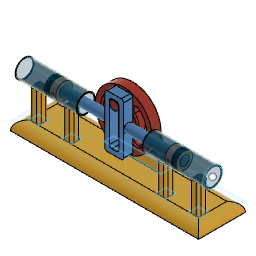
Scotch Yoke Mechanism (Autodesk Fusion 360 design; units mm, degrees)
Autodesk Fusion 360 part; units mm, degrees
sketch "base" plane through (0, 0, 0) normal (0, 0, 1) x (1, 0, 0) in component "Holder"
  line L0 (100, 0) -> (100, 25)
  line L1 (100, 0) -> (100, -25)
  line L2 (-100, 0) -> (-100, 25)
  line L3 (-100, 0) -> (-100, -25)
  line L4 (-100, 25) -> (100, 25)
  line L5 (-100, -25) -> (100, -25)
  dimension "d1" = 100
  dimension "d5" = 50
  constraint vertical L0
  constraint perpendicular L0 L4
  constraint perpendicular L1 L5
  measures "d1" distance of origin L0.start
  measures "d5" distance of L4 L5
extrude "Extrude1" add sketch "base" along normal blind 10 makes body 1 in component "Holder"
sketch "holders" plane through (0, 0, 10) normal (0, 0, 1) x (-1, 0, 0) in component "Holder"
  line L0 (100, -25) -> (100, 25)
  line L1 (100, 25) -> (-100, 25)
  line L2 (-100, 25) -> (-100, -25)
  line L3 (-100, -25) -> (100, -25)
  line L4 (30, -15) -> (-30, -15)
  line L5 (-30, -15) -> (-30, -5)
  line L6 (-30, -5) -> (30, -5)
  line L7 (30, -5) -> (30, -15)
  line L8 (90, 14.85) -> (80, 14.85)
  line L9 (80, 14.85) -> (80, 5)
  line L10 (80, 5) -> (90, 5)
  line L11 (55, 14.85) -> (45, 14.85)
  line L12 (45, 14.85) -> (45, 5)
  line L13 (45, 5) -> (55, 5)
  line L14 (55, 5) -> (55, 14.85)
  line L15 (-80, 14.85) -> (-90, 14.85)
  line L16 (-90, 5) -> (-80, 5)
  line L17 (-80, 5) -> (-80, 14.85)
  line L18 (-45, 14.85) -> (-55, 14.85)
  line L19 (-55, 14.85) -> (-55, 5)
  line L20 (-55, 5) -> (-45, 5)
  line L21 (-45, 5) -> (-45, 14.85)
  line L22 (-90, 5) -> (-90, 14.85)
  line L23 (90, 5) -> (90, 14.85)
  dimension "d8" = 60
  dimension "d9" = 10
  constraint horizontal L4
  constraint vertical L5
  constraint horizontal L6
  constraint vertical L7
  constraint horizontal L8
  constraint vertical L9
  constraint horizontal L10
  constraint horizontal L11
  constraint vertical L12
  constraint horizontal L13
  constraint vertical L14
  constraint horizontal L15
  constraint horizontal L16
  constraint vertical L17
  constraint horizontal L18
  constraint vertical L19
  constraint horizontal L20
  constraint vertical L21
  measures "d8" distance of L4.start L4.end
  measures "d9" distance of L4.start L6.end
extrude "Extrude2" add sketch "holders" along normal blind 40 contours L8 L9 L10 L23 | L11 L12 L13 L14 | L15 L16 L17 L22 | L18 L19 L20 L21 bodies 1 in component "Holder"
extrude "Extrude4" cut sketch "holders" against normal blind 40 contours L4 L5 L6 L7 bodies 1 in component "Holder"
sketch "crank holder" plane through (0, 0, 0) normal (0, 1, 0) x (1, 0, 0) in component "Crank holder"
  line L0 (29.85, -10.4) -> (15, -50)
  line L1 (-29.85, -10.4) -> (-15, -50)
  arc A0 (-15, -50) -> (15, -50) centre (0, -50) ccw
  line L2 (29.85, -10.4) -> (29.85, 0)
  line L3 (29.85, 0) -> (-29.85, 0)
  line L4 (-29.85, 0) -> (-29.85, -10.4)
  constraint vertical L2
  constraint perpendicular L2 L3
  constraint perpendicular L3 L4
extrude "Extrude1'" add sketch "crank holder" along normal blind 10 from surface at 5 separate body makes body 2 in component "Crank holder"
move_face "OffsetFaces1" offset -0.3 1 faces at (5, 5, 23.6) on bodies 2 in component "Crank holder"
sketch "circle" plane through (0, 5.3, 0) normal (0, -1, 0) x (1, 0, 0) in component "Crank holder"
  line L0 (29.85, 0) -> (29.85, 10.4)
  line L1 (29.85, 10.4) -> (15, 50)
  arc A0 (15, 50) -> (-15, 50) centre (0, 50) ccw
  line L2 (-15, 50) -> (-29.85, 10.4)
  line L3 (-29.85, 10.4) -> (-29.85, 0)
  line L4 (-29.85, 0) -> (29.85, 0)
  circle A1 centre (0, 50) radius 5
  dimension "d21" = 10
  constraint concentric A0 A1
  measures "d21" diameter of A1
extrude "Extrude2'" add sketch "circle" along normal blind 10 contours A1 bodies 2 in component "Crank holder"
move_face "OffsetFaces2" offset -0.3 1 faces at (4.9938, -1.3667, 49.7508) on bodies 2 in component "Crank holder"
sketch "crank" plane through (0, 5.3, 0) normal (0, -1, 0) x (1, 0, 0) in component "Crank"
  circle A0 centre (0, 50) radius 4.7
  line L0 (29.85, 0) -> (29.85, 10.4)
  line L1 (29.85, 10.4) -> (15, 50)
  arc A1 (15, 50) -> (-15, 50) centre (0, 50) ccw
  line L2 (-15, 50) -> (-29.85, 10.4)
  line L3 (-29.85, 10.4) -> (-29.85, 0)
  line L4 (-29.85, 0) -> (29.85, 0)
  circle A2 centre (0, 50) radius 30
  circle A3 centre (0, 50) radius 5
  circle A4 centre (0, 68) radius 4.7
  arc A5 (16.2474, 66.2795) -> (10.5962, 60.617) centre (13.4218, 63.4482) ccw
  arc A6 (-10.5962, 60.617) -> (-16.2474, 66.2795) centre (-13.4218, 63.4482) ccw
  arc A7 (-16.2474, 33.7205) -> (-10.5962, 39.383) centre (-13.4218, 36.5518) ccw
  arc A8 (10.5962, 39.383) -> (16.2474, 33.7205) centre (13.4218, 36.5518) ccw
  line L5 (0, 55) -> (0, 54.7)
  line L6 (0, 45.3) -> (0, 45)
  arc A9 (-10.5962, 60.617) -> (-10.5962, 39.383) centre (0, 50) ccw
  arc A10 (10.5962, 39.383) -> (10.5962, 60.617) centre (0, 50) ccw
  arc A11 (-16.2474, 66.2795) -> (-16.2474, 33.7205) centre (0, 50) ccw
  arc A12 (16.2474, 33.7205) -> (16.2474, 66.2795) centre (0, 50) ccw
  constraint concentric A0 A2
  constraint concentric A0 A3
  constraint concentric A2 A9
  constraint coincident L1.end A9
  constraint concentric A3 A11
  constraint tangent A5 A11
  constraint vertical L5
  constraint symmetric A5 A6 L5
  constraint tangent A5 A9
  constraint tangent A6 A9
  constraint tangent A7 A9
  constraint coincident A1 A5.end
  constraint coincident A1 A6.start
  constraint coincident A8.end A11
  constraint coincident A8.start A9
  constraint coincident A0 L5.end
  constraint coincident A0 L6.start
  constraint collinear L5 L6
  constraint concentric A9 A10
  constraint concentric A11 A12
extrude "Extrude1''" add sketch "crank" along normal blind 10 separate body contours L1 A1 L2 A2 A4 A7 A8 A9 A10 A11 A12 | L1 A1 L2 A2 A4 A5 A6 A11 A12 | A1 A4 | A1 A4 makes body 3 in component "Crank"
extrude "Extrude2''" add sketch "crank" along normal blind 20 contours A1 A4 | A1 A4 bodies 3 in component "Crank"
move_face "OffsetFaces1'" offset -0.3 1 faces at (0.7473, 5.3, 29.9985) on bodies 3 in component "Crank"
sketch "piston" plane through (0, 0, 0) normal (1, 0, 0) x (0, 1, 0) in component "Right piston"
  circle A0 centre (-10, 50) radius 10
  circle A1 centre (-10, 50) radius 9
  constraint concentric A0 A1
extrude "Extrude1'''" add sketch "piston" along normal blind 65 from surface at 35 separate body makes body 4 in component "Right piston"
sketch "connecting rod" plane through (0, -4.7, 0) normal (0, -1, 0) x (1, 0, 0) in component "Connecting rod"
  circle A0 centre (0, 68) radius 4.7
  circle A1 centre (0, 50) radius 5
  arc A2 (-10.5962, 60.617) -> (-16.2474, 66.2795) centre (-13.4218, 63.4482) ccw
  arc A3 (-10.5962, 60.617) -> (-10.5962, 39.383) centre (0, 50) ccw
  arc A4 (-16.2474, 33.7205) -> (-10.5962, 39.383) centre (-13.4218, 36.5518) ccw
  arc A5 (-16.2474, 66.2795) -> (-16.2474, 33.7205) centre (0, 50) ccw
  arc A6 (10.5962, 39.383) -> (16.2474, 33.7205) centre (13.4218, 36.5518) ccw
  arc A7 (10.5962, 39.383) -> (10.5962, 60.617) centre (0, 50) ccw
  arc A8 (16.2474, 66.2795) -> (10.5962, 60.617) centre (13.4218, 63.4482) ccw
  arc A9 (16.2474, 33.7205) -> (16.2474, 66.2795) centre (0, 50) ccw
  circle A10 centre (0, 50) radius 30
  line L0 (-7.5, 78) -> (7.5, 78)
  line L1 (10, 75.5) -> (10, 24.5)
  line L2 (-10, 24.5) -> (-10, 75.5)
  line L3 (-5, 29.5) -> (-5, 70.5)
  line L4 (-2.5, 73) -> (2.5, 73)
  line L5 (5, 70.5) -> (5, 29.5)
  line L6 (-2.5, 27) -> (2.5, 27)
  line L7 (-7.5, 22) -> (7.5, 22)
  arc A11 (-2.5, 73) -> (-5, 70.5) centre (-2.5, 70.5) ccw
  arc A12 (5, 70.5) -> (2.5, 73) centre (2.5, 70.5) ccw
  arc A13 (-7.5, 78) -> (-10, 75.5) centre (-7.5, 75.5) ccw
  arc A14 (10, 75.5) -> (7.5, 78) centre (7.5, 75.5) ccw
  arc A15 (-5, 29.5) -> (-2.5, 27) centre (-2.5, 29.5) ccw
  arc A16 (2.5, 27) -> (5, 29.5) centre (2.5, 29.5) ccw
  arc A17 (-10, 24.5) -> (-7.5, 22) centre (-7.5, 24.5) ccw
  arc A18 (7.5, 22) -> (10, 24.5) centre (7.5, 24.5) ccw
  point P0 (-10, 78)
  point P1 (10, 78)
  dimension "d33" = 20
  dimension "d36" = 2.5
  constraint horizontal L0
  constraint vertical L1
  constraint vertical L2
  constraint parallel L2 L3
  constraint parallel L0 L4
  constraint parallel L1 L5
  constraint tangent L3 A11
  constraint tangent L4 A11
  constraint tangent L4 A12
  constraint tangent L5 A12
  constraint equal A11 A12
  constraint coincident P0 L2
  constraint coincident P0 L0
  constraint tangent L2 A13
  constraint tangent L0 A13
  constraint equal A11 A13
  constraint coincident P1 L0
  constraint coincident P1 L1
  constraint tangent L0 A14
  constraint tangent L1 A14
  constraint equal A11 A14
  constraint tangent L3 A15
  constraint tangent L6 A15
  constraint equal A11 A15
  constraint tangent L5 A16
  constraint tangent L6 A16
  constraint equal A11 A16
  constraint tangent L2 A17
  constraint tangent L7 A17
  constraint equal A11 A17
  constraint tangent L1 A18
  constraint tangent L7 A18
  constraint equal A11 A18
  measures "d33" distance of P0 P1
  measures "d36" radius of A11
extrude "Extrude1''''" add sketch "connecting rod" along normal blind 9.7 from surface at 0.3 separate body contours A2 L2 | A2 A4 A6 A8 L0 L1 L2 L7 A13 A14 A17 A18 | A4 L2 | A8 L1 | A6 L1 makes body 5 in component "Connecting rod"
sketch "tube" plane through (0, 0, 0) normal (1, 0, 0) x (0, 1, 0) in component "Connecting rod"
  circle A0 centre (-9.85, 50) radius 4.85
  dimension "d40" = 9.7
  measures "d40" diameter of A0
extrude "Extrude2'''" add sketch "tube" along normal blind 60 from surface at 10 bodies 5 in component "Connecting rod"
extrude "Extrude3" add sketch "tube" against normal blind 60 from surface at -10 bodies 5 in component "Connecting rod"
sketch "deleting useless material" plane through (100, 0, 0) normal (1, 0, 0) x (0, 1, 0) in component "Holder"
  circle A0 centre (-10, 50) radius 9
  circle A1 centre (-10, 50) radius 10
  circle A2 centre (-10, 50) radius 10
  constraint concentric A0 A2
extrude "Extrude5" cut sketch "deleting useless material" against normal blind 65 contours A0 | A1 A2 bodies 1 in component "Holder"
extrude "Extrude6" cut sketch "deleting useless material" against normal blind 70 from surface at -132 contours A0 | A1 A2 bodies 1 in component "Holder"
sketch "piston (2)" plane through (0, 0, 0) normal (1, 0, 0) x (0, 1, 0) in component "Left piston"
  circle A0 centre (-10, 50) radius 10
  circle A1 centre (-10, 50) radius 9
  constraint concentric A0 A1
extrude "Extrude1'''''" add sketch "piston (2)" against normal blind 65 from surface at -35 separate body makes body 6 in component "Left piston"
sketch "rightt" plane through (70, 0, 0) normal (1, 0, 0) x (0, 1, 0) in component "Connecting rod"
  circle A0 centre (-9.85, 50) radius 4.85
  circle A1 centre (-10, 50) radius 8.85
  dimension "d55" = 17.7
  measures "d55" diameter of A1
sketch "left" plane through (-70, 0, 0) normal (-1, 0, 0) x (0, -1, 0) in component "Connecting rod"
  circle A0 centre (9.85, 50) radius 4.85
  circle A1 centre (10, 50) radius 8.85
  dimension "d56" = 17.7
  measures "d56" diameter of A1
extrude "Extrude4'" add sketch "rightt" against normal blind 12 separate body makes body 7 in component "Connecting rod"
extrude "Extrude5'" add sketch "left" against normal blind 12 separate body makes body 8 in component "Connecting rod"
fillet "Fillet1" radius 1.5 4 edges at (-15, -4.7, 50) (-10.5906, -4.7, 33.7261) (-23, -4.7, 50) (-10.5906, -4.7, 66.2739) on bodies 3 in component "Crank"
fillet "Fillet2" radius 1.5 4 edges at (10.5906, -4.7, 33.7261) (15, -4.7, 50) (10.5906, -4.7, 66.2739) (23, -4.7, 50) on bodies 3 in component "Crank"
fillet "Fillet3" radius 1.5 4 edges at (10.5906, 5, 66.2739) (23, 5, 50) (10.5906, 5, 33.7261) (15, 5, 50) on bodies 3 in component "Crank"
fillet "Fillet4" radius 1.5 4 edges at (-23, 5, 50) (-10.5906, 5, 66.2739) (-15, 5, 50) (-10.5906, 5, 33.7261) on bodies 3 in component "Crank"
fillet "Fillet1'" radius 10 4 edges at (0, -25, 10) (100, 0, 10) (0, 25, 10) (-100, 0, 10) on bodies 1 in component "Holder"
fillet "Fillet2'" radius 2.5 14 edges at (55, -14.85, 25.6274) (90, -14.85, 25.6274) (45, -14.85, 25.6274) (55, -5, 25.6699) (90, -5, 25.6699) (-45, -14.85, 25.6274) (-45, -5, 25.6699) (-80, -14.85, 25.6274) (-80, -5, 25.6699) (-90, -14.85, 25.6274) (-90, -5, 25.6699) (-55, -5, 25.6699) (80, -5, 25.6699) (45, -5, 25.6699) on bodies 1 in component "Holder"
fillet "Fillet3'" radius 2.5 1 edges at (80, -14.85, 25.6274) on bodies 1 in component "Holder"
fillet "Fillet4'" radius 2.5 1 edges at (-55, -14.85, 25.6274) on bodies 1 in component "Holder"
sketch "circular model" plane through (70, 0, 0) normal (1, 0, 0) x (0, 1, 0) in component "Connecting rod"
  circle A0 centre (-10, 50) radius 8.85
  circle A1 centre (-10, 50) radius 8.85
  circle A2 centre (-10, 50) radius 7.5
  circle A3 centre (-9.85, 50) radius 4.85
  dimension "d98" = 15
  dimension "d99" = 17.7
  constraint concentric A0 A1
  constraint concentric A1 A2
  measures "d98" diameter of A2
  measures "d99" diameter of A1
extrude "Extrude6'" cut sketch "circular model" against normal blind 0.8 from surface at -1.2 contours A0 A1 bodies 7 8 5 in component "Connecting rod"
extrude "Extrude7" cut sketch "circular model" against normal blind 0.8 from surface at -2.8 contours A0 A1 bodies 7 5 8 in component "Connecting rod"
extrude "Extrude8" cut sketch "circular model" against normal blind 0.8 from surface at -4.4 contours A0 A1 bodies 8 7 5 in component "Connecting rod"
sketch "right circle" plane through (0, 0, 0) normal (0, 1, 0) x (1, 0, 0) in component "Connecting rod"
  circle A0 centre (61.4, -50) radius 1.1
extrude "Extrude9" cut sketch "right circle" against normal blind 4 from the near side of the face at (60.2667, -1.161, 49.5589) on bodies 7 bodies 5 7 8 in component "Connecting rod"
extrude "Extrude10" cut sketch "right circle" along normal blind 4 from the near side of the face at (61.3987, -1.4058, 47.8877) on bodies 7 bodies 5 8 7 in component "Connecting rod"
extrude "Extrude11" cut sketch "circular model" along normal blind 0.8 from surface at -138.8 contours A0 A1 bodies 8 5 7 in component "Connecting rod"
extrude "Extrude12" cut sketch "circular model" against normal blind 0.8 from surface at -136.4 contours A0 A1 bodies 8 5 7 in component "Connecting rod"
extrude "Extrude13" cut sketch "circular model" against normal blind 0.8 from surface at -134.8 contours A0 A1 bodies 8 5 7 in component "Connecting rod"
sketch "left circle" plane through (0, 0, 0) normal (0, 1, 0) x (1, 0, 0) in component "Connecting rod"
  circle A0 centre (-61.4, -50) radius 1.1
  dimension "d110" = 2.2
  measures "d110" diameter of A0
extrude "Extrude14" cut sketch "left circle" against normal blind 4 from the near side of the face at (-62.5333, -18.839, 49.5589) on bodies 8 bodies 8 5 7 in component "Connecting rod"
extrude "Extrude15" cut sketch "left circle" along normal blind 4 from the near side of the face at (-61.4016, -1.4058, 47.8877) on bodies 8 bodies 5 8 7 in component "Connecting rod"
move_face "OffsetFaces1''" offset -0.3 1 faces at (63.1642, -5.3374, 51.7773) on bodies 7 in component "Connecting rod"
move_face "OffsetFaces2'" offset -0.3 1 faces at (-63.1576, -5.3376, 48.2222) on bodies 8 in component "Connecting rod"
move_face "OffsetFaces1'''" offset -0.3 4 faces at (-83.3333, -10.7385, 40.0273) (-48.3333, -10.7385, 40.0273) (51.6667, -10.7385, 40.0273) (86.6667, -10.7385, 40.0273) on bodies 1 in component "Holder"
component "Holder" placed x (1, 0, 0) y (0, 1, 0) z (0, 0, 1) at (0, 0, 0)
component "Crank holder" placed x (1, 0, 0) y (0, 1, 0) z (0, 0, 1) at (0, 0, 0)
component "Crank" placed x (1, 0, 0) y (0, 1, 0) z (0, 0, 1) at (0, 0, 0)
component "Right piston" placed x (1, 0, 0) y (0, 1, 0) z (0, 0, 1) at (0, 0, 0)
component "Connecting rod" placed x (1, 0, 0) y (0, 1, 0) z (0, 0, 1) at (0, 0, 0)
component "Left piston" placed x (1, 0, 0) y (0, 1, 0) z (0, 0, 1) at (0, 0, 0)
named bodies: "Holder", "Crank holder", "Crank", "Right piston", "Connecting rod", "Left piston", "Right tube", "Left tube"
